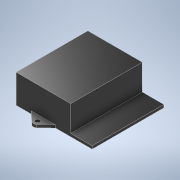
# Autodesk Inventor part: 25W_1224_5V
Saved by Autodesk Inventor 2021 (Build 250183000, 183)
## iProperties
Created: 2022-01-13
Part Number: 25W_1224_5V
Material: Generic
Document SubType Name: Modeling
Designer: Jorian Brusind
Density: 1 g/cm^3
Appearance: Glossy - Black
Author: Jorian Brusind
Autodesk Inventor part; units mm, degrees
ref_plane "YZ Plane" through (0, 0, 0) normal (1, 0, 0) x (0, 1, 0)
ref_plane "XZ Plane" through (0, 0, 0) normal (0, 1, 0) x (-1, 0, 0)
sketch "Sketch1" plane through (0, 0, 0) normal (0, 1, 0) x (-1, 0, 0)
  line L0 (0, 0) -> (38, 0)
  line L1 (38, 0) -> (38, -50)
  line L2 (38, -50) -> (0, -50)
  line L3 (0, -50) -> (0, 0)
  dimension "d0" = 38
  dimension "d1" = 50
  constraints: 8 end point, 2 parallel, 1 horizontal, 1 perpendicular
  measures "d0" distance of L1.end L2.end
  measures "d1" distance of L0.end L1.end
extrude "Extrusion1" add sketch "Sketch1" along normal blind 20
sketch "Sketch2" plane through (0, 0, 0) normal (0, -1, 0) x (1, 0, 0)
  line L0 (0, 0) -> (0, -50) projected
  line L1 (0, 0) -> (15, 0)
  line L2 (15, 0) -> (15, -50)
  line L3 (15, -50) -> (0, -50)
  line L4 (0, -50) -> (0, 0)
  dimension "d4" = 15
  dimension "d5" = 50
  constraints: 8 end point, 2 parallel, 1 horizontal, 1 perpendicular
  measures "d4" distance of L2.end L3.end
  measures "d5" distance of L1.end L2.end
extrude "Extrusion2" add sketch "Sketch2" against normal blind 2
sketch "Sketch3" plane through (0, 0, 0) normal (0, -1, 0) x (1, 0, 0)
  line L0 (-38, 0) -> (0, 0) projected
  line L1 (-19, 0) -> (-19, 7)
  line L2 (-19, 0) -> (-19, 4)
  line L3 (-19, 0) -> (-10.5, 0)
  line L4 (-19, 0) -> (-27.5, 0)
  circle A0 centre (-19, 4) radius 1.5
  circle A1 centre (-19, 4) radius 3
  line L5 (-10.5, 0) -> (-17.5, 6.5981)
  line L6 (-27.5, 0) -> (-20.5, 6.5981)
  dimension "d8" = 7
  dimension "d9" = 4
  dimension "d10" = 8.5
  dimension "d11" = 8.5
  dimension "d12" = 3
  dimension "d13" = 6.5981
  dimension "d14" = 6.5981
  constraints: 12 end point, 3 point on circle, 3 point on line, 2 centre point, 2 coincident, 1 midpoint, 1 vertical
  measures "d8" distance of L1.start L1.end
  measures "d9" distance of L1.start L2.end
  measures "d10" distance of L1.start L3.end
  measures "d11" distance of L1.start L4.end
  measures "d12" diameter of A0
  measures "d13" vertical distance of L4.end L6.end
  measures "d14" vertical distance of L3.end L5.end
extrude "Extrusion3" add sketch "Sketch3" against normal blind 2 contours L6 A1 L1 L0 | L1 A1 L5 L0 | L6 A1 L1 A0 | L1 A0 A1 L5
ref_plane "Work Plane1" through (-38, 20, -25) normal (0, 0, 1) x (1, 0, 0)
mirror "Mirror1" about plane through (-38, 20, -25) normal (0, 0, 1) of "Extrusion3"
body "Solid1"
